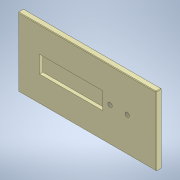
# Autodesk Inventor part: podstwa
Saved by Autodesk Inventor 2021 (Build 250183000, 183)
## iProperties
Created: 2021-11-16
Part Number: podstwa
Material: MDF — płyta pilśniowa o średniej gęstości
Document SubType Name: Modeling
Designer: wojwo
Density: 0.8 g/cm^3
Appearance: Gładki — popielaty
Author: wojwo
Autodesk Inventor part; units mm, degrees
ref_plane "YZ Plane" through (0, 0, 0) normal (1, 0, 0) x (0, 1, 0)
ref_plane "XZ Plane" through (0, 0, 0) normal (0, 1, 0) x (-1, 0, 0)
ref_plane "XY Plane" through (0, 0, 0) normal (0, 0, 1) x (1, 0, 0)
sketch "Szkic1" plane through (0, 0, 0) normal (0, 0, 1) x (1, 0, 0)
  line L0 (-60, -30) -> (60, -30)
  line L1 (60, -30) -> (60, 30)
  line L2 (60, 30) -> (-60, 30)
  line L3 (-60, 30) -> (-60, -30)
  line L4 (-60, -30) -> (60, 30) construction
  line L5 (60, -30) -> (-60, 30) construction
  point P0 (0, 0)
  dimension "d0" = 120
  dimension "d1" = 60
  constraints: 12 end point, 2 midpoint, 2 parallel, 1 horizontal, 1 perpendicular
  measures "d0" distance of L2.end L1.end
  measures "d1" distance of L1.end L0.end
extrude "Wyciągnięcie proste1" add sketch "Szkic1" against normal blind 5
sketch "Szkic2" plane through (0, 0, 0) normal (0, 0, 1) x (1, 0, 0)
  circle A0 centre (-35, 0) radius 2.5 projected
  circle A1 centre (-20, 0) radius 2.5 projected
  circle A2 centre (20, 0) radius 2 projected
  circle A3 centre (35, 0) radius 2 projected
  line L0 (-39.7, -6.05) -> (-39.7, 6.05) projected
  line L1 (39.7, -6.05) -> (-39.7, -6.05) projected
  line L2 (39.7, 6.05) -> (39.7, -6.05) projected
  line L3 (-39.7, 6.05) -> (39.7, 6.05) projected
  line L4 (-41.5, 7.5) -> (13.5, 7.5)
  line L5 (13.5, 7.5) -> (13.5, -7.5)
  line L6 (13.5, -7.5) -> (-41.5, -7.5)
  line L7 (-41.5, -7.5) -> (-41.5, 7.5)
  line L8 (-41.5, 7.5) -> (13.5, -7.5) construction
  line L9 (13.5, 7.5) -> (-41.5, -7.5) construction
  point P0 (0, 0)
  point P1 (-14, 0)
  dimension "d4" = 55
  dimension "d5" = 15
  dimension "d6" = 14
  constraints: 12 end point, 2 midpoint, 2 parallel, 1 horizontal, 1 perpendicular
  measures "d4" distance of L5.end L6.end
  measures "d5" distance of L4.end L5.end
  measures "d6" distance of point (0, 0) point (-14, 0)
extrude "Wyciągnięcie proste2" cut sketch "Szkic2" against normal blind 3 contours A0 | A1 | L1 L5 L6 L7 L4 L3 L0 | L0 L3 L5 L1
sketch "Szkic3" plane through (0, 0, 0) normal (0, 0, 1) x (1, 0, 0)
  circle A0 centre (35, 0) radius 2 projected
  circle A1 centre (20, 0) radius 2 projected
  point P0 (0, 0)
extrude "Wyciągnięcie proste3" cut sketch "Szkic3" against normal through all
thread "Gwint1" size "M4x0.7" class "6H" standard "ANSI Metric M Profile" full length
thread "Gwint2" size "M4x0.7" class "6H" standard "ANSI Metric M Profile" full length
chamfer "Faza2" distance 0.5 angle 45 9 edges at (60, 30, -2.5) (0, 30, 0) (0, 30, -5) (60, 0, 0) (60, 0, -5) (0, -30, 0) (0, -30, -5) (-60, 0, 0) (-60, 0, -5)
chamfer "Faza3" distance 2 angle 45 2 edges at (18, 0, -5) (33, 0, -5)
